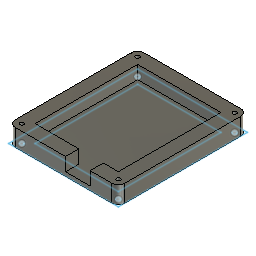
prvpad_bot (Autodesk Fusion 360 design; units mm, degrees)
part number: 2026-03-04-21-57-17-026
Autodesk Fusion 360 part; units mm, degrees
sketch "Sketch1" plane through (0, 0, 0) normal (0, 0, 1) x (1, 0, 0)
  line L0 (-15.6254, 36.106) -> (47.1246, 36.106)
  line L1 (47.1246, 36.106) -> (47.1246, -41.1843)
  line L2 (47.1246, -41.1843) -> (-15.6254, -41.1843)
  line L3 (-15.6254, -41.1843) -> (-15.6254, 36.106)
  line L4 (-25.6254, 46.106) -> (57.1246, 46.106)
  line L5 (57.1246, 46.106) -> (57.1246, -51.1843)
  line L6 (57.1246, -51.1843) -> (-25.6254, -51.1843)
  line L7 (-25.6254, -51.1843) -> (-25.6254, 46.106)
  circle A0 centre (-20.6254, 41.106) radius 1.45
  circle A1 centre (52.5, 41.106) radius 1.45
  circle A2 centre (52.1246, -46.1843) radius 1.45
  circle A3 centre (-20.6254, -46.1843) radius 1.45
  dimension "d1" = 77.2903
  dimension "d2" = 62.75
  dimension "d3" = 10
  dimension "d4" = 10
  dimension "d5" = 10
  dimension "d6" = 10
  dimension "d7" = 2.9
  dimension "d8" = 5
  dimension "d9" = 5
  dimension "d10" = 2.9
  dimension "d11" = 2.9
  dimension "d12" = 2.9
  dimension "d13" = 5
  dimension "d14" = 5
  dimension "d15" = 5
  dimension "d16" = 5
  dimension "d17" = 5
  constraint horizontal L0
  constraint vertical L1
  constraint horizontal L2
  constraint vertical L3
  constraint horizontal L4
  constraint vertical L5
  constraint horizontal L6
  constraint vertical L7
  measures "d1" distance of L0 L2
  measures "d2" distance of L1 L3
  measures "d3" distance of L2 L6
  measures "d4" distance of L1 L5
  measures "d5" distance of L0 L4
  measures "d6" distance of L3 L7
  measures "d7" diameter of A0
  measures "d8" distance of L4 A0.centre
  measures "d9" distance of L7 A0.centre
  measures "d10" diameter of A3
  measures "d11" diameter of A2
  measures "d12" diameter of A1
  measures "d13" distance of L4 A1.centre
  measures "d14" distance of L5 A2.centre
  measures "d15" distance of L6 A2.centre
  measures "d16" distance of L6 A3.centre
  measures "d17" distance of L7 A3.centre
extrude "Extrude3" add sketch "Sketch1" along normal blind 3 contours L0 L1 L2 L3
extrude "Extrude4" add sketch "Sketch1" along normal blind 13
sketch "Sketch3" plane through (0, -51.1843, 0) normal (0, -1, 0) x (1, 0, 0)
  line L0 (-25.6254, 0) -> (57.1246, 0)
  line L1 (57.1246, 0) -> (57.1246, 13)
  line L2 (57.1246, 13) -> (-25.6254, 13)
  line L3 (-25.6254, 13) -> (-25.6254, 0)
  line L4 (17.2996, 13) -> (35.7996, 13)
  line L5 (35.7996, 13) -> (35.7996, 3)
  line L6 (35.7996, 3) -> (17.2996, 3)
  line L7 (17.2996, 3) -> (17.2996, 13)
  dimension "d26" = 21.325
  dimension "d27" = 18.5
  constraint horizontal L4
  constraint vertical L5
  constraint horizontal L6
  constraint vertical L7
  constraint coincident L2 L4.start
  measures "d26" distance of L1 L5
  measures "d27" distance of L5 L7
extrude "Extrude5" cut sketch "Sketch3" against normal blind 13 contours L2 L4 L5 L6 L7
fillet "Fillet1" radius 5 4 edges at (57.1246, 46.106, 6.5) (-25.6254, 46.106, 6.5) (-25.6254, -51.1843, 6.5) (57.1246, -51.1843, 6.5)
extrude "Extrude1" [suppressed]
extrude "Extrude2" [suppressed]
